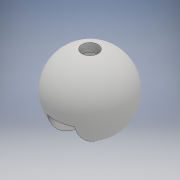
# Autodesk Inventor part: Нар
Saved by Autodesk Inventor 2017 (Build 210142000, 142)
## iProperties
Part Number: Нар
Material: Типовые
Document SubType Name: Modeling
Designer: 2000
Density: 1 g/cm^3
Appearance: По умолчанию
Author: 2000
Autodesk Inventor part; units mm, degrees
ref_plane "YZ Plane" through (0, 0, 0) normal (1, 0, 0) x (0, 1, 0)
ref_plane "XZ Plane" through (0, 0, 0) normal (0, 1, 0) x (-1, 0, 0)
ref_plane "XY Plane" through (0, 0, 0) normal (0, 0, 1) x (1, 0, 0)
sketch "Эскиз1" plane through (0, 0, 0) normal (0, 0, 1) x (1, 0, 0)
  arc A0 (0, -35) -> (0, 35) centre (0, 0) ccw
  arc A1 (0, -45) -> (0, 45) centre (0, 0) ccw
  line L0 (0, 45) -> (0, 35)
  line L1 (0, -45) -> (0, -35)
  line L2 (0, -63) -> (0, 63) projected
  dimension "d0" = 35
  dimension "d1" = 45
  constraints: 4 end point, 4 point on circle, 4 vertical alignment, 2 centre point, 2 coincident, 1 collinear, 1 vertical
  measures "d0" radius of A0
  measures "d1" radius of A1
revolve "Вращение1" add sketch "Эскиз1" angle 360 about axis through (0, -10, 0) along (0, 1, 0) contours A0 L0 A1 L1
sketch "Эскиз2" plane through (0, 0, 0) normal (0, 0, 1) x (1, 0, 0)
  circle A0 centre (0, 0) radius 10
  dimension "d3" = 20
  constraints: 1 centre point, 1 coincident
  measures "d3" diameter of A0
extrude "Выдавливание1" cut sketch "Эскиз2" along normal through all
sketch "Эскиз3" plane through (0, 0, 0) normal (0, 1, 0) x (-1, 0, 0)
  line L0 (10, -45) -> (-20, -45)
  line L1 (-20, -45) -> (-20, -10)
  line L2 (-20, -10) -> (10, -10)
  line L3 (10, -10) -> (10, -45)
  line L4 (-10, 43.8748) -> (10, 43.8748) projected
  line L5 (-10, 43.8748) -> (10, 43.8748) projected
  arc A0 (-10, 43.8748) -> (10, 43.8748) centre (0, 0) ccw projected
  arc A1 (-10, 43.8748) -> (10, 43.8748) centre (0, 0) ccw projected
  dimension "d6" = 30
  dimension "d7" = 10
  dimension "d8" = 10
  constraints: 8 end point, 2 parallel, 1 horizontal, 1 perpendicular, 1 tangent
  measures "d6" distance of L0.start L0.end
  measures "d7" distance from line of A0.centre L2
  measures "d8" distance from line of A0.centre L3
extrude "Выдавливание2" cut sketch "Эскиз3" along normal through all both and the other way through all contours L0 A0 L3 | L0 L1 A0 | A0 L1 L2 L3
